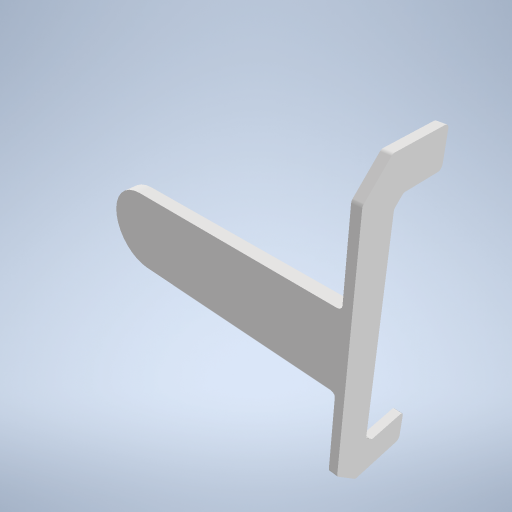
# Autodesk Inventor part: Holder
Saved by Autodesk Inventor 2023 (Build 270158000, 158)
## iProperties
Created: 2023-09-22
Part Number: Holder
Material: Generic
Document SubType Name: Modeling
Designer: vlada
Density: 1 g/cm^3
Appearance: Default
Author: vlada
Autodesk Inventor part; units mm, degrees
ref_plane "YZ Plane" through (0, 0, 0) normal (1, 0, 0) x (0, 1, 0)
ref_plane "XZ Plane" through (0, 0, 0) normal (0, 1, 0) x (-1, 0, 0)
ref_plane "XY Plane" through (0, 0, 0) normal (0, 0, 1) x (1, 0, 0)
sketch "Sketch1" plane through (0, 0, 0) normal (0, 0, 1) x (1, 0, 0)
  line L0 (-8.5494, 35.2005) -> (51.4506, 35.2005)
  line L1 (51.4506, 35.2005) -> (51.4506, 53.2005)
  line L2 (51.4506, 53.2005) -> (-8.5494, 53.2005)
  line L3 (-8.5494, 53.2005) -> (-8.5494, 35.2005)
  point P0 (0, 0)
  dimension "d0" = 18
  dimension "d1" = 60
  constraints: 8 end point, 2 parallel, 1 horizontal, 1 perpendicular
  measures "d0" distance of L2.end L0.start
  measures "d1" distance of L1.end L2.end
extrude "Extrusion1" add sketch "Sketch1" along normal blind 3
sketch "Sketch2" plane through (0, 0, 0) normal (0, 0, -1) x (-1, 0, 0)
  circle A0 centre (-0.4506, 44.2005) radius 4
  line L0 (-0.4506, 44.2005) -> (8.5494, 44.2005) construction
  line L1 (8.5494, 53.2005) -> (8.5494, 35.2005) projected
  line L2 (-0.4506, 44.2005) -> (-0.4506, 35.2005) construction
  line L3 (8.5494, 35.2005) -> (-51.4506, 35.2005) projected
  line L4 (-0.4506, 44.2005) -> (-0.4506, 53.2005) construction
  line L5 (-51.4506, 53.2005) -> (8.5494, 53.2005) projected
  point P0 (0, 0)
  dimension "d4" = 8
  constraints: 6 end point, 3 point on line, 2 equal length, 1 centre point, 1 horizontal, 1 midpoint, 1 perpendicular
  measures "d4" diameter of A0
extrude "Extrusion2" add sketch "Sketch2" along normal blind 5
sketch "Sketch4" plane through (0.4506, 44.2005, -5) normal (0, 0, -1) x (-1, 0, 0)
  circle A0 centre (0, 0) radius 4 projected
  circle A1 centre (0, 0) radius 4
  line L0 (4, -3.1231) -> (4, 2.6998) construction
  point P0 (0.4506, -44.2005)
  constraints: 2 end point, 1 centre point, 1 coincident, 1 vertical
revolve "Revolution1" [suppressed]
sketch "Sketch5" plane through (0.2094, 44.2005, -3.3681) normal (-0.3420201, 0, -0.9396926) x (-0.9396926, 0, 0.3420201)
  ellipse E0 centre (0, 0) end of major axis (0, -4) minor radius 4
  point P0 (1.3487, -44.2005)
  constraints: 2 other
extrude "Extrusion3" [suppressed]
fillet "Fillet1" radius 9 2 edges at (-8.5494, 35.2005, 1.5) (-8.5494, 53.2005, 1.5)
sketch "Sketch6" plane through (51.4506, 35.2005, 0) normal (1, 0, 0) x (0, 0, -1)
  line L0 (-3, 44) -> (17, 44)
  line L1 (17, -26) -> (-3, -26)
  line L2 (-3, -26) -> (-3, 44)
  line L3 (-3, 0) -> (-3, 18) projected
  line L4 (0, 0) -> (-3, 0) projected
  line L5 (0, 0) -> (-3, -26) construction
  line L6 (0, 18) -> (-3, 18) projected
  line L7 (0, 18) -> (-3, 44) construction
  line L8 (17, 44) -> (17, 36)
  line L9 (17, 36) -> (5, 36)
  line L10 (5, 36) -> (5, -18)
  line L11 (5, -18) -> (17, -18)
  line L12 (17, -18) -> (17, -26)
  point P0 (0, -35.2005)
  dimension "d11" = 70
  dimension "d12" = 0
  dimension "d15" = 20
  dimension "d16" = 8
  dimension "d17" = 8
  dimension "d18" = 8
  dimension "d19" = 20
  constraints: 20 end point, 3 perpendicular, 2 horizontal, 1 equal length, 1 parallel, 1 vertical
  measures "d11" distance of L0.end L1.start
  measures "d12" distance between parallel lines of L3 L2
  measures "d15" distance of L0.start L0.end
  measures "d16" distance of L0.end L8.end
  measures "d17" distance of L11.end L1.start
  measures "d18" distance between parallel lines of L10 L2
  measures "d19" distance of L1.start L1.end
extrude "Extrusion4" add sketch "Sketch6" along normal blind 2
chamfer "Chamfer1" distance 6 angle 45 2 edges at (52.4506, 79.2005, 3) (52.4506, 9.2005, 3)
chamfer "Chamfer2" distance 2 angle 45 2 edges at (52.4506, 17.2005, -5) (52.4506, 71.2005, -5)
fillet "Fillet3" radius 1 15 edges at (52.4506, 17.2005, -17) (52.4506, 9.2005, -17) (52.4506, 79.2005, -17) (52.4506, 71.2005, -17) (52.4506, 71.2005, -7) (52.4506, 69.2005, -5) (52.4506, 19.2005, -5) (52.4506, 17.2005, -7) (52.4506, 79.2005, -3) (52.4506, 73.2005, 3) (52.4506, 9.2005, -3) (52.4506, 15.2005, 3) (51.4506, 53.2005, 1.5) (51.4506, 44.2005, 0) (51.4506, 35.2005, 1.5)
fillet "Fillet4" radius 1 1 edges at (4.4506, 44.2005, -5)
equation "\"d17\" = d16"
equation "\"d18\" = d16"
equation "\"d19\" = d15"
body "Solid1"
